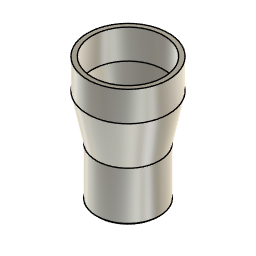
adapter_festool_vaccum_cleaner (Autodesk Fusion 360 design; units mm, degrees)
Autodesk Fusion 360 part; units mm, degrees
sketch "adapter_side" plane through (0, 0, 0) normal (0, 0, 1) x (1, 0, 0)
  circle A0 centre (0, 0) radius 21
  dimension "d33" = 42
  constraint coincident A0.centre origin
  measures "d33" diameter of A0
extrude "Extrude2" add sketch "adapter_side" along normal blind 33 makes body 1
ref_plane "WorkPlane2" through (0, 0, 63) normal (0, 0, 1) x (1, 0, 0)
sketch "bandsaw_side" plane through (0, 0, 63) normal (0, 0, 1) x (1, 0, 0)
  circle A0 centre (0, 0) radius 27
  dimension "d38" = 54
  constraint coincident A0.centre origin
  measures "d38" diameter of A0
extrude "Extrude3" add sketch "bandsaw_side" along normal blind 20 separate body makes body 2
loft "Loft3" add section 1 face at (-5.9246, 2.0633, 33) section 2 face at (4.9388, -0.7444, 63) on bodies 1 2 bodies 1 2
shell "Shell1" thickness 3 removed faces 2 at (-5.9246, 2.0633, 0) at (4.9388, -0.7444, 83) on bodies 1
sketch "pins" plane through (0, 0, 0) normal (0, 1, 0) x (1, 0, 0)
  line L0 (18, 0) -> (18, -33.2971)
  line L1 (-18, -33.2971) -> (-18, 0)
  line L2 (18, -14) -> (16.25, -14)
  line L3 (16.25, -14) -> (16.25, -6)
  line L4 (16.25, -6) -> (18, -6)
  line L5 (18, -6) -> (18, -14)
  dimension "d42" = 1.75
  dimension "d43" = 8
  dimension "d44" = 6
  constraint horizontal L2
  constraint vertical L3
  constraint horizontal L4
  constraint vertical L5
  constraint coincident L0 L2.start
  measures "d42" distance of L2.start L2.end
  measures "d43" distance of L2.start L4.end
  measures "d44" distance of L0.start L4.end
revolve "Revolve3" add sketch "pins" angle 44 about axis through (0, 0, 1.75) along (0, 0, 1) separate body makes body 3
chamfer "Chamfer2" distance 1.75 angle 45 4 edges at (15.0667, 6.0874, 14) (16.25, 0, 10) (15.0667, 6.0874, 6) (11.6893, 11.2882, 10) on bodies 3
pattern_circular "C-Pattern2" count 3 over 360 about axis through (0, 0, 1.75) along (0, 0, 1) of bodies 3 makes body 4 at (-16.2088, 7.8279, 8.6667) makes body 5 at (-5.4959, -17.1405, 8.6667)
chamfer "Chamfer3" distance 1 angle 45 2 edges at (-19.5789, -7.5939, 0) (-16.7819, -6.5091, 0) on bodies 1
equation "d_adapter_inside = 36 mm" comment "inner diameter of adapter"
equation "t = 3 mm" comment "Thikness of adapter wall"
equation "t_pin = 1.75 mm" comment "Thickness of pins"
equation "l_pin = 8 mm"
equation "s_bottom_pin = 6 mm" comment "space from bottom to pin"
equation "s_top_pin = 19 mm" comment "space from top to pin"
equation "chamfer_bottom = 1 mm" comment "chamfer at bottom of adapter"
equation "l_adapter = s_bottom_pin + l_pin + s_top_pin"
equation "a_pin = 44 deg" comment "Angle of pin"
equation "d_bandsaw_inside = 54 mm"
equation "l_bandsaw = 20 mm"
equation "d33 = d_adapter_inside + 2 * t"
equation "d34 = l_adapter"
equation "l_adapter_to_bandsaw = 30 mm"
equation "d37 = l_adapter_to_bandsaw"
equation "d38 = d_bandsaw_inside"
equation "d39 = l_bandsaw"
equation "d42 = t_pin"
equation "d43 = l_pin"
equation "d44 = s_bottom_pin"
equation "d45 = a_pin"
equation "d46 = chamfer_pin"
equation "d49 = chamfer_bottom"
equation "chamfer_pin = t_pin"
named bodies: "Shell", "Pin", "Pin (1)", "Pin (2)"
